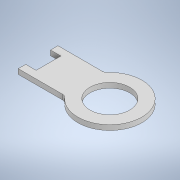
# Autodesk Inventor part: kkekey
Saved by Autodesk Inventor 2022 (Build 260153000, 153)
## iProperties
Created: 2024-10-04
Part Number: kkekey
Material: Типовые
Document SubType Name: Modeling
Designer: korsh624
Density: 1 g/cm^3
Appearance: По умолчанию
Author: korsh624
Autodesk Inventor part; units mm, degrees
ref_plane "YZ Plane" through (0, 0, 0) normal (1, 0, 0) x (0, 1, 0)
ref_plane "XZ Plane" through (0, 0, 0) normal (0, 1, 0) x (-1, 0, 0)
ref_plane "XY Plane" through (0, 0, 0) normal (0, 0, 1) x (1, 0, 0)
sketch "Эскиз1" plane through (0, 0, 0) normal (0, 1, 0) x (-1, 0, 0)
  line L0 (0, 0) -> (4.2, 0)
  line L1 (4.2, 0) -> (4.2, -3)
  line L2 (4.2, -3) -> (0, -3)
  line L3 (0, -3) -> (0, -13)
  line L4 (4.2, -13) -> (0, -13)
  line L5 (4.2, -13) -> (4.2, -16)
  line L6 (4.2, -16) -> (0, -16)
  line L7 (0, -16) -> (-9.7125, -16)
  line L8 (-9.7125, -16) -> (-9.7125, 0)
  line L9 (-9.7125, 0) -> (4.2, 0)
  dimension "d0" = 4.2
  dimension "d1" = 10
  dimension "d2" = 3
  dimension "d3" = 3
  constraints: 20 end point, 6 perpendicular, 5 point on line, 1 collinear, 1 horizontal
  measures "d0" distance of L1.end L2.end
  measures "d1" distance of L2.end L3.end
  measures "d2" distance of L0.end L1.end
  measures "d3" distance of L4.start L5.end
extrude "Выдавливание1" add sketch "Эскиз1" along normal blind 2
sketch "Эскиз2" plane through (0, 2, 0) normal (0, 1, 0) x (1, 0, 0)
  line L0 (9.7125, 0) -> (9.7125, 16) projected
  line L1 (9.7125, 8) -> (24.7125, 8)
  circle A0 centre (24.7125, 8) radius 12.9007
  circle A1 centre (24.7125, 8) radius 8
  line L2 (9.7125, 16) -> (-4.2, 16) projected
  line L3 (9.7125, 16) -> (14.5918, 16)
  line L4 (-4.2, 0) -> (9.7125, 0) projected
  line L5 (9.7125, 0) -> (14.5918, 0)
  point P0 (0, 0)
  dimension "d6" = 15
  constraints: 6 end point, 2 centre point, 2 coincident, 2 point on circle, 1 collinear, 1 horizontal, 1 midpoint
  measures "d6" distance of L1.start L1.end
extrude "Выдавливание2" add sketch "Эскиз2" against normal blind 2
fillet "Сопряжение1" radius 2 2 edges at (14.5918, 1, -16) (14.5918, 1, 0)
